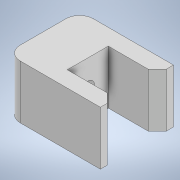
# Autodesk Inventor part: Part feature intro
Saved by Autodesk Inventor 2020 (Build 240152000, 152)
## iProperties
Created: 2019-02-24
Part Number: Part feature intro
Material: Generic
Document SubType Name: Modeling
Designer: John Helfen
Density: 1 g/cm^3
Appearance: Default
Author: John Helfen
Autodesk Inventor part; units mm, degrees
ref_plane "YZ Plane" through (0, 0, 0) normal (1, 0, 0) x (0, 1, 0)
ref_plane "XZ Plane" through (0, 0, 0) normal (0, 1, 0) x (-1, 0, 0)
ref_plane "XY Plane" through (0, 0, 0) normal (0, 0, 1) x (1, 0, 0)
sketch "Sketch1" plane through (0, 0, 0) normal (0, 0, 1) x (1, 0, 0)
  line L0 (0, 0) -> (32.6151, 0)
  line L1 (32.6151, 0) -> (32.6151, 18.65)
  line L2 (32.6151, 18.65) -> (0, 18.65)
  line L3 (0, 18.65) -> (0, 0)
  constraints: 8 end point, 2 parallel, 1 horizontal, 1 perpendicular
extrude "Extrusion1" add sketch "Sketch1" along normal blind 25.4
sketch "Sketch2" plane through (0, 18.65, 0) normal (0, 1, 0) x (1, 0, 0)
  line L0 (32.6151, 0) -> (32.6151, -25.4) projected
  line L1 (32.6151, -19.8922) -> (15.5994, -19.8922)
  line L2 (15.5994, -19.8922) -> (15.5994, -5.6439)
  line L3 (15.5994, -5.6439) -> (32.6151, -5.6439)
  line L4 (32.6151, -5.6439) -> (32.6151, -19.8922)
  line L5 (15.5994, -5.6439) -> (15.5994, -0.1361) construction
  line L6 (32.6151, -25.4) -> (0, -25.4) projected
  line L7 (15.5994, -25.4) -> (15.5994, -19.8922) construction
  point P0 (0, 0)
  constraints: 12 end point, 2 parallel, 2 perpendicular, 2 point on line, 1 collinear, 1 horizontal, 1 vertical
extrude "Extrusion2" cut sketch "Sketch2" against normal through all
fillet "Fillet1" radius 4.7625 2 edges at (0, 9.325, 25.4) (0, 9.325, 0)
chamfer "Chamfer1" distance 3.175 angle 45 2 edges at (32.6151, 9.325, 19.8922) (32.6151, 9.325, 5.6439)
sketch "Sketch3" plane through (15.5994, 18.65, 19.8922) normal (1, 0, 0) x (0, 0, -1)
  line L0 (14.2482, 0) -> (14.2482, -18.65) projected
  line L1 (14.2482, -18.65) -> (0, 0) construction
  point P0 (19.8922, -18.65)
  point P1 (7.1241, -9.325)
  constraints: 2 end point, 1 midpoint
hole "Hole1" at (15.5994, 9.325, 12.768) direction (-1, 0, 0) diameter 3.175 end through all countersink diameter 4.7625 countersink angle 82
body "Solid1"
